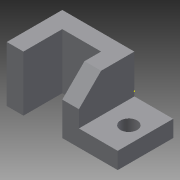
# Autodesk Inventor part: 2-4
Saved by Autodesk Inventor 2015 (Build 190159000, 159)
## iProperties
Created: 2015-08-31
Part Number: 2-4
Material: Generic
Document SubType Name: Modeling
Designer: Brandon
Density: 1 g/cm^3
Appearance: Default
Author: Brandon
Autodesk Inventor part; units mm, degrees
ref_plane "YZ Plane" through (0, 0, 0) normal (1, 0, 0) x (0, 1, 0)
ref_plane "XZ Plane" through (0, 0, 0) normal (0, 1, 0) x (-1, 0, 0)
ref_plane "XY Plane" through (0, 0, 0) normal (0, 0, 1) x (1, 0, 0)
sketch "Sketch1" plane through (0, 0, 0) normal (0, 0, 1) x (1, 0, 0)
  line L0 (11.7764, -24.2743) -> (75.2764, -24.2743)
  line L1 (75.2764, -24.2743) -> (75.2764, -5.2243)
  line L2 (75.2764, -5.2243) -> (30.8264, -5.2243)
  line L3 (30.8264, -5.2243) -> (30.8264, 39.2257)
  line L4 (30.8264, 39.2257) -> (11.7764, 39.2257)
  line L5 (11.7764, 39.2257) -> (11.7764, -24.2743)
  point P0 (0, 0)
  dimension "d0" = 19.05
  dimension "d1" = 63.5
  dimension "d2" = 63.5
  dimension "d3" = 19.05
  constraints: 12 end point, 5 perpendicular, 1 horizontal
  measures "d0" distance of L3.end L4.end
  measures "d1" distance of L4.end L0.start
  measures "d2" distance of L0.start L0.end
  measures "d3" distance of L0.end L1.end
extrude "Extrusion1" add sketch "Sketch1" along normal blind 63.5
sketch "Sketch2" plane through (11.7764, 39.2257, 0) normal (0, 1, 0) x (1, 0, 0)
  line L0 (0, 0) -> (-63.5, 0)
  line L1 (-63.5, 0) -> (-63.5, -63.5)
  line L2 (-63.5, -63.5) -> (-44.45, -63.5)
  line L3 (0, 0) -> (0, -19.05)
  line L4 (0, -19.05) -> (-44.45, -19.05)
  line L5 (-44.45, -19.05) -> (-44.45, -63.5)
  line L6 (0, 0) -> (0, -63.5) projected
  point P0 (-11.7764, 0)
  dimension "d6" = 63.5
  dimension "d7" = 63.5
  dimension "d8" = 19.05
  dimension "d9" = 19.05
  dimension "d10" = 0
  dimension "d11" = 0
  constraints: 12 end point, 4 perpendicular, 1 horizontal, 1 vertical
  measures "d6" distance of L0.start L0.end
  measures "d7" distance of L0.end L1.end
  measures "d8" distance of L1.end L2.end
  measures "d9" distance of L0.start L3.end
  measures "d10" distance between parallel lines of L6 L3
  measures "d11" vertical distance of L0.start point (-11.776, 0)
extrude "Extrusion2" add sketch "Sketch2" against normal blind 63.5
sketch "Sketch3" plane through (30.8264, -5.2243, 0) normal (0, 1, 0) x (1, 0, 0)
  circle A0 centre (25.4, -31.75) radius 9.525
  line L0 (44.45, 0) -> (44.45, -63.5) projected
  line L1 (44.45, 0) -> (0, 0) projected
  point P0 (-30.8264, 0)
  dimension "d14" = 19.05
  dimension "d15" = 19.05
  dimension "d16" = 31.75
  constraints: 1 centre point
  measures "d14" diameter of A0
  measures "d15" distance from line of L0 A0.centre
  measures "d16" distance from line of L1 A0.centre
extrude "Extrusion3" cut sketch "Sketch3" against normal through all
sketch "Sketch4" plane through (30.8264, -5.2243, 0) normal (1, 0, 0) x (0, 0, -1)
  point P0 (0, 5.2243)
sketch "Sketch5" plane through (30.8264, -5.2243, 0) normal (1, 0, 0) x (0, 0, -1)
  point P0 (0, 5.2243)
sketch "Sketch6" plane through (30.8264, -5.2243, 0) normal (1, 0, 0) x (0, 0, -1)
  line L0 (-63.5, 44.45) -> (-38.1, 44.45)
  line L1 (0, 44.45) -> (-63.5, 44.45) projected
  line L2 (-38.1, 44.45) -> (-63.5, 19.05)
  line L3 (-63.5, 19.05) -> (-63.5, 44.45)
  point P0 (0, 5.2243)
  dimension "d19" = 25.4
  dimension "d20" = 45
  constraints: 6 end point, 1 perpendicular, 1 point on line
  measures "d19" distance of L0.start L0.end
  measures "d20" angle of L0 L2
extrude "Extrusion4" cut sketch "Sketch6" against normal up to next
body "Solid1"
